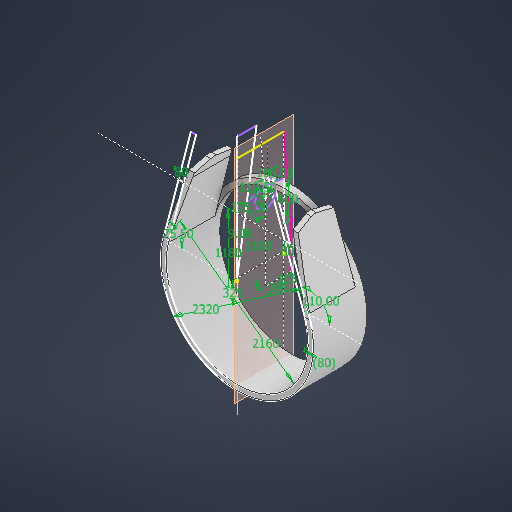
# Autodesk Inventor part: Part2
Saved by Autodesk Inventor 2026.2 (Build 302298000, 298)
## iProperties
Created: 2025-12-11
Part Number: Part2
Material: Generic
Document SubType Name: Modeling
Designer: bubim
Density: 1 g/cm^3
Appearance: Default
Author: bubim
Autodesk Inventor part; units mm, degrees
ref_plane "YZ Plane" through (0, 0, 0) normal (1, 0, 0) x (0, 1, 0)
ref_plane "XZ Plane" through (0, 0, 0) normal (0, 1, 0) x (-1, 0, 0)
ref_plane "XY Plane" through (0, 0, 0) normal (0, 0, 1) x (1, 0, 0)
sketch "Sketch1" plane through (0, 0, 0) normal (0, 0, 1) x (1, 0, 0)
  arc A0 (-1040.213506, 290.440805) -> (1016.915041, 363.708398) centre (0, 0) ccw
  arc A1 (-1123.051263, 290.440805) -> (1090.04344, 396.743366) centre (0, 0) ccw
  line L0 (-1123.051263, 290.440805) -> (-892.995613, 1180)
  line L1 (-1123.051263, 290.440805) -> (-204.225292, 290.440805) construction
  line L2 (1090.04344, 396.743366) -> (804.96134, 1180)
  line L3 (1090.04344, 396.743366) -> (1923.56774, 396.743366) construction
  line L4 (0, 0) -> (0, 1180) construction
  line L5 (0, 1180) -> (1900.808505, 1180) construction
  line L6 (1900.808505, 1180) -> (-2124.970927, 1180) construction
  line L7 (804.96134, 1180) -> (724.96134, 1180) construction
  line L8 (804.96134, 1180) -> (724.96134, 1180)
  line L9 (724.96134, 1180) -> (1016.915041, 363.708398)
  line L10 (-892.995613, 1180) -> (-812.995613, 1180)
  line L11 (-812.995613, 1180) -> (-1046.3284, 267.575934)
  line L12 (-892.995613, 1180) -> (-706.077385, 1902.759157)
  line L13 (-706.077385, 1902.759157) -> (-626.077385, 1902.759157)
  line L14 (-626.077385, 1902.759157) -> (-812.995613, 1180)
  line L15 (724.96134, 1180) -> (461.89852, 1902.759157)
  line L16 (461.89852, 1902.759157) -> (541.89852, 1902.759157)
  line L17 (541.89852, 1902.759157) -> (804.96134, 1180)
  dimension "d1" = 2160
  dimension "d2" = 2320
  dimension "d4" = 80
  dimension "d5" = 75.5
  dimension "d6" = 110
  dimension "d7" = 1180
  dimension "d8" = 80
  dimension "d9" = 80
  constraints: 36 end point, 6 point on line, 5 point on circle, 4 horizontal, 4 tangent, 3 parallel, 2 centre point, 2 collinear, 2 equal length, 1 coincident, 1 perpendicular, 1 vertical, 1 other
  measures "d1" diameter of A0
  measures "d2" diameter of A1
  measures "d4" radial gap between concentric circles of A1 A0
  measures "d5" angle of L1 L0
  measures "d6" angle of L3 L2
  measures "d7" distance of L4.start L4.end
  measures "d8" distance of L2.end L7.end
  measures "d9" distance of L0.end L10.end
extrude "Extrusion1" add sketch "Sketch1" against normal blind 710
ref_plane "Work Plane1" through (0, 0, 0) normal (1, 0, 0) x (0, 1, 0)
sketch "Sketch2" plane through (0, 0, 0) normal (1, 0, 0) x (0, 1, 0)
  line L0 (0, 0) -> (325, 0) construction
  line L1 (396.743366, 0) -> (-1160, 0) construction
  line L2 (325, 0) -> (325, -710) construction
  line L3 (-1160, -710) -> (396.743366, -710) construction
  line L4 (325, 0) -> (2190.73627, -295.503595)
  line L5 (325, 0) -> (2213.992907, 0) construction
  line L6 (2190.73627, -295.503595) -> (2190.73627, 0)
  line L7 (1902.759157, 0) -> (1902.759157, -710)
  line L8 (2190.73627, 0) -> (325, 0)
  line L9 (0, -815) -> (0, -430) construction
  line L10 (0, -430) -> (1180, -430) construction
  line L11 (1180, -430) -> (2009.151875, -357.458611) construction
  line L12 (1180, -430) -> (1334.410178, -416.49086) construction
  arc A0 (1180, -416.49086) -> (1180, -430) centre (1257.205089, -423.24543) ccw
  line L13 (1334.410178, -416.49086) -> (1425.077731, -416.49086) construction
  circle A1 centre (1180, -430) radius 155
  line L14 (1325.184189, -375.717856) -> (1238.82339, -144.735406)
  line L15 (1325.184189, -375.717856) -> (1634.970705, -375.717856) construction
  line L16 (1332.404511, -458.246506) -> (1285.744759, -710)
  line L17 (1332.404511, -458.246506) -> (1864.039818, -458.246506) construction
  line L18 (0, -815) -> (0, -710) construction
  line L19 (0, -710) -> (1902.759157, -710) construction
  line L20 (1285.744759, -710) -> (685.744759, -710)
  line L21 (685.744759, -710) -> (685.744759, -815)
  line L22 (685.744759, -815) -> (0, -815)
  line L23 (685.744759, -815) -> (1902.759157, -815)
  point P0 (290.440805, 0)
  point P1 (396.743366, -710)
  point P2 (290.440805, -710)
  point P3 (1902.759157, -249.892501)
  dimension "d13" = 325
  dimension "d14" = 9
  dimension "d17" = 385
  dimension "d18" = 1180
  dimension "d19" = 175
  dimension "d20" = 155
  dimension "d22" = 110.5
  dimension "d23" = 100.5
  dimension "d24" = 105
  dimension "d25" = 600
  constraints: 42 end point, 8 point on line, 5 horizontal, 5 perpendicular, 4 point on circle, 2 centre point, 2 coincident, 2 tangent, 1 collinear, 1 equal length, 1 midpoint, 1 parallel, 1 vertical, 4 other
  measures "d13" distance of L0.start L0.end
  measures "d14" angle of L4 L5
  measures "d17" distance of L9.start L9.end
  measures "d18" distance of L9.end L10.end
  measures "d19" angle of L11 L10
  measures "d20" distance of L12.end L10.end
  measures "d22" angle of L15 L14
  measures "d23" angle of L16 L17
  measures "d24" distance of L9.start L18.end
  measures "d25" distance of L16.end L20.end
sketch "Sketch2 outline for Extrusion2" plane through (0, 0, 0) normal (1, 0, 0) x (0, 1, 0)
  line L0 (2190.73627, -295.503595) -> (2190.73627, 0)
  line L1 (2190.73627, 0) -> (325, 0)
  line L2 (325, 0) -> (1238.82339, -144.735406)
  line L3 (1238.82339, -144.735406) -> (1325.184189, -375.717856)
  arc A0 (1325.184189, -375.717856) -> (1332.404511, -458.246506) centre (1180, -430) cw
  line L4 (1332.404511, -458.246506) -> (1285.744759, -710)
  line L5 (1285.744759, -710) -> (685.744759, -710)
  line L6 (685.744759, -710) -> (685.744759, -815)
  line L7 (685.744759, -815) -> (1902.759157, -710)
  line L8 (1902.759157, -710) -> (1902.759157, -249.892501)
  line L9 (1902.759157, -249.892501) -> (2190.73627, -295.503595)
extrude "Extrusion2" cut sketch "Sketch2 outline for Extrusion2" along normal through all both and the other way through all
sketch "Sketch5" plane through (0, 0, -710) normal (0, 0, -1) x (-1, 0, 0)
  circle A0 centre (0, 0) radius 1080
  circle A1 centre (0, 0) radius 1160
  constraints: 2 centre point, 2 coincident
extrude "Extrusion3" add sketch "Sketch5" along normal blind 105
body "Solid1"
